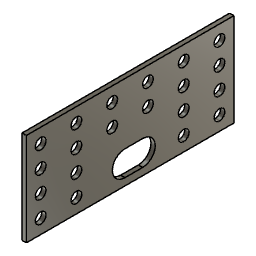
electronic_box_assembly v3 (Autodesk Fusion 360 archive; units mm, degrees)
design "plate_4"
Autodesk Fusion 360 part; units mm, degrees
sketch "Sketch1" plane through (0, 0, 0) normal (1, 0, 0) x (0, 1, 0)
  line L0 (0, 0) -> (290.2, 0)
  line L1 (290.2, 0) -> (290.2, 130)
  line L2 (290.2, 130) -> (0, 130)
  line L3 (0, 130) -> (0, 0)
  dimension "d1" = 290.2
  dimension "d2" = 130
  constraint horizontal L0
  constraint vertical L1
  constraint horizontal L2
  constraint vertical L3
  constraint coincident L0.start L3.end
  measures "d1" distance of L0.start L0.end
  measures "d2" distance of L0.start L2.end
extrude "Extrude1" add sketch "Sketch1" against normal blind 6
sketch "Sketch2" plane through (0, 0, 0) normal (1, 0, 0) x (0, 1, 0)
  line L0 (0, 130) -> (0, 0)
  line L1 (0, 0) -> (290.2, 0)
  line L2 (290.2, 0) -> (290.2, 130)
  line L3 (290.2, 130) -> (0, 130)
  line L4 (162.7, 45) -> (137.7, 45)
  arc A0 (137.7, 45) -> (137.7, 10) centre (137.7, 27.5) ccw
  line L5 (137.7, 10) -> (162.7, 10)
  arc A1 (162.7, 10) -> (162.7, 45) centre (162.7, 27.5) ccw
  line L6 (180.2, 27.5) -> (120.2, 27.5) construction
  circle A2 centre (20, 110) radius 7.5
  circle A3 centre (70, 110) radius 7.5
  circle A4 centre (120, 110) radius 7.5
  circle A5 centre (170, 110) radius 7.5
  circle A6 centre (220, 110) radius 7.5
  circle A7 centre (270, 110) radius 7.5
  circle A8 centre (20, 80) radius 7.5
  circle A9 centre (70, 80) radius 7.5
  circle A10 centre (120, 80) radius 7.5
  circle A11 centre (170, 80) radius 7.5
  circle A12 centre (220, 80) radius 7.5
  circle A13 centre (270, 80) radius 7.5
  circle A14 centre (20, 50) radius 7.5
  circle A15 centre (70, 50) radius 7.5
  circle A16 centre (220, 50) radius 7.5
  circle A17 centre (270, 50) radius 7.5
  circle A18 centre (20, 20) radius 7.5
  circle A19 centre (70, 20) radius 7.5
  circle A20 centre (220, 20) radius 7.5
  circle A21 centre (270, 20) radius 7.5
  dimension "d5" = 35
  dimension "d6" = 110
  dimension "d7" = 10
  dimension "d8" = 15
  dimension "d9" = 20
  dimension "d10" = 20
  dimension "d13" = 250
  dimension "d14" = -90
  constraint tangent L4 A0
  constraint tangent A0 L5
  constraint parallel L4 L5
  constraint tangent L5 A1
  constraint tangent L4 A1
  constraint midpoint A1 L6.start
  constraint midpoint A0 L6.end
  constraint horizontal L6
  measures "d5" diameter of A0
  measures "d6" distance of L2 L6.start
  measures "d7" distance of L1 L5
  measures "d8" diameter of A2
  measures "d9" distance of L3 A2.centre
  measures "d10" distance of L0 A2.centre
extrude "Extrude2" cut sketch "Sketch2" against normal up to surface (6 mm away) contours L4 A0 L5 A1 | A2 | A3 | A4 | A5 | A6 | A7 | A8 | A9 | A10 | A11 | A12 | A13 | A14 | A15 | A16 | A17 | A18 | A19 | A20 | A21

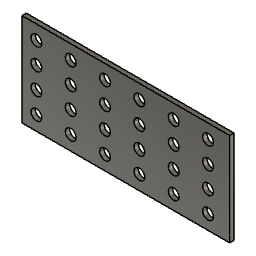
design "plate_2"
Autodesk Fusion 360 part; units mm, degrees
sketch "Sketch1" plane through (0, 0, 0) normal (0, 1, 0) x (1, 0, 0)
  line L0 (0, 0) -> (290.2, 0)
  line L1 (290.2, 0) -> (290.2, -130)
  line L2 (290.2, -130) -> (0, -130)
  line L3 (0, -130) -> (0, 0)
  dimension "d1" = 290.2
  dimension "d2" = 130
  constraint horizontal L0
  constraint vertical L1
  constraint horizontal L2
  constraint vertical L3
  constraint coincident L0.start L3.end
  measures "d1" distance of L0.start L0.end
  measures "d2" distance of L0.start L2.end
extrude "Extrude1" add sketch "Sketch1" against normal blind 6
sketch "Sketch2" plane through (0, -6, 0) normal (0, -1, 0) x (1, 0, 0)
  line L0 (290.2, 130) -> (0, 130)
  line L1 (0, 130) -> (0, 0)
  line L2 (0, 0) -> (290.2, 0)
  line L3 (290.2, 0) -> (290.2, 130)
  circle A0 centre (20, 110) radius 7.5
  circle A1 centre (68, 110) radius 7.5
  circle A2 centre (116, 110) radius 7.5
  circle A3 centre (164, 110) radius 7.5
  circle A4 centre (212, 110) radius 7.5
  circle A5 centre (260, 110) radius 7.5
  circle A6 centre (20, 80) radius 7.5
  circle A7 centre (68, 80) radius 7.5
  circle A8 centre (116, 80) radius 7.5
  circle A9 centre (164, 80) radius 7.5
  circle A10 centre (212, 80) radius 7.5
  circle A11 centre (260, 80) radius 7.5
  circle A12 centre (20, 50) radius 7.5
  circle A13 centre (68, 50) radius 7.5
  circle A14 centre (116, 50) radius 7.5
  circle A15 centre (164, 50) radius 7.5
  circle A16 centre (212, 50) radius 7.5
  circle A17 centre (260, 50) radius 7.5
  circle A18 centre (20, 20) radius 7.5
  circle A19 centre (68, 20) radius 7.5
  circle A20 centre (116, 20) radius 7.5
  circle A21 centre (164, 20) radius 7.5
  circle A22 centre (212, 20) radius 7.5
  circle A23 centre (260, 20) radius 7.5
  dimension "d5" = 15
  dimension "d6" = 20
  dimension "d7" = 20
  dimension "d10" = 240
  dimension "d11" = -90
  measures "d5" diameter of A0
  measures "d6" distance of L0 A0.centre
  measures "d7" distance of L1 A0.centre
extrude "Extrude2" cut sketch "Sketch2" against normal up to surface (6 mm away) contours A0 | A1 | A2 | A3 | A4 | A5 | A6 | A7 | A8 | A9 | A10 | A11 | A12 | A13 | A14 | A15 | A16 | A17 | A18 | A19 | A20 | A21 | A22 | A23

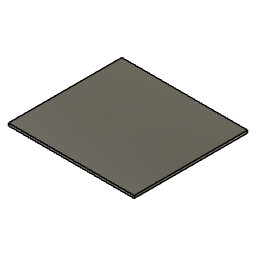
design "base_plate"
Autodesk Fusion 360 part; units mm, degrees
sketch "Sketch1" plane through (0, 0, 0) normal (0, 0, 1) x (1, 0, 0)
  line L0 (0, 0) -> (302.2, 0)
  line L1 (302.2, 0) -> (302.2, 272.2)
  line L2 (302.2, 272.2) -> (0, 272.2)
  line L3 (0, 272.2) -> (0, 0)
  dimension "d1" = 302.2
  dimension "d2" = 272.2
  constraint horizontal L0
  constraint vertical L1
  constraint horizontal L2
  constraint vertical L3
  constraint coincident L0.start L3.end
  measures "d1" distance of L0.start L0.end
  measures "d2" distance of L0 L2
extrude "Extrude1" add sketch "Sketch1" against normal blind 6

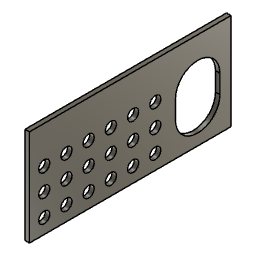
design "plate_1"
Autodesk Fusion 360 part; units mm, degrees
sketch "Sketch1" plane through (0, 0, 0) normal (1, 0, 0) x (0, 1, 0)
  line L0 (0, 0) -> (272.2, 0)
  line L1 (272.2, 0) -> (272.2, 130)
  line L2 (272.2, 130) -> (0, 130)
  line L3 (0, 130) -> (0, 0)
  dimension "d1" = 272.2
  dimension "d2" = 130
  constraint horizontal L0
  constraint vertical L1
  constraint horizontal L2
  constraint vertical L3
  constraint coincident L0.start L3.end
  measures "d1" distance of L0.start L0.end
  measures "d2" distance of L0.start L2.end
extrude "Extrude1" add sketch "Sketch1" against normal blind 6
sketch "Sketch2" plane through (0, 0, 0) normal (1, 0, 0) x (0, 1, 0)
  line L0 (0, 130) -> (0, 0)
  line L1 (0, 0) -> (272.2, 0)
  line L2 (272.2, 0) -> (272.2, 130)
  line L3 (272.2, 130) -> (0, 130)
  line L4 (257.2, 45) -> (257.2, 70)
  arc A0 (257.2, 70) -> (197.2, 70) centre (227.2, 70) ccw
  line L5 (197.2, 70) -> (197.2, 45)
  arc A1 (197.2, 45) -> (257.2, 45) centre (227.2, 45) ccw
  line L6 (227.2, 15) -> (227.2, 100) construction
  circle A2 centre (20, 80) radius 7.5
  circle A3 centre (50, 80) radius 7.5
  circle A4 centre (80, 80) radius 7.5
  circle A5 centre (110, 80) radius 7.5
  circle A6 centre (140, 80) radius 7.5
  circle A7 centre (170, 80) radius 7.5
  circle A8 centre (20, 50) radius 7.5
  circle A9 centre (50, 50) radius 7.5
  circle A10 centre (80, 50) radius 7.5
  circle A11 centre (110, 50) radius 7.5
  circle A12 centre (140, 50) radius 7.5
  circle A13 centre (170, 50) radius 7.5
  circle A14 centre (20, 20) radius 7.5
  circle A15 centre (50, 20) radius 7.5
  circle A16 centre (80, 20) radius 7.5
  circle A17 centre (110, 20) radius 7.5
  circle A18 centre (140, 20) radius 7.5
  circle A19 centre (170, 20) radius 7.5
  dimension "d5" = 60
  dimension "d6" = 15
  dimension "d7" = 15
  constraint tangent L4 A0
  constraint tangent A0 L5
  constraint parallel L4 L5
  constraint tangent L5 A1
  constraint tangent L4 A1
  constraint midpoint A1 L6.start
  constraint midpoint A0 L6.end
  constraint perpendicular L3 L6
  measures "d5" diameter of A0
  measures "d6" distance of L1 L6.start
  measures "d7" distance of L2 L4
extrude "Extrude2" cut sketch "Sketch2" against normal up to surface (6 mm away) contours L4 A0 L5 A1 | A2 | A3 | A4 | A5 | A6 | A7 | A8 | A9 | A10 | A11 | A12 | A13 | A14 | A15 | A16 | A17 | A18 | A19

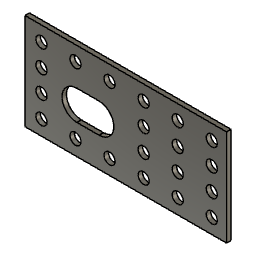
design "plate_3"
Autodesk Fusion 360 part; units mm, degrees
sketch "Sketch1" plane through (0, 0, 0) normal (0, 1, 0) x (1, 0, 0)
  line L0 (0, 0) -> (272.2, 0)
  line L1 (272.2, 0) -> (272.2, -130)
  line L2 (272.2, -130) -> (0, -130)
  line L3 (0, -130) -> (0, 0)
  dimension "d1" = 272.2
  dimension "d2" = 130
  constraint horizontal L0
  constraint vertical L1
  constraint horizontal L2
  constraint vertical L3
  constraint coincident L0.start L3.end
  measures "d1" distance of L0.start L0.end
  measures "d2" distance of L0.start L2.end
extrude "Extrude1" add sketch "Sketch1" against normal blind 6
sketch "Sketch2" plane through (0, -6, 0) normal (0, -1, 0) x (1, 0, 0)
  line L0 (272.2, 130) -> (0, 130)
  line L1 (0, 130) -> (0, 0)
  line L2 (0, 0) -> (272.2, 0)
  line L3 (272.2, 0) -> (272.2, 130)
  line L4 (70, 40) -> (100, 40)
  arc A0 (100, 40) -> (100, 80) centre (100, 60) ccw
  line L5 (100, 80) -> (70, 80)
  arc A1 (70, 80) -> (70, 40) centre (70, 60) ccw
  line L6 (50, 60) -> (120, 60) construction
  circle A2 centre (252.2, 110) radius 7.5
  circle A3 centre (206.2, 110) radius 7.5
  circle A4 centre (160.2, 110) radius 7.5
  circle A5 centre (114.2, 110) radius 7.5
  circle A6 centre (68.2, 110) radius 7.5
  circle A7 centre (252.2, 80) radius 7.5
  circle A8 centre (206.2, 80) radius 7.5
  circle A9 centre (252.2, 50) radius 7.5
  circle A10 centre (206.2, 50) radius 7.5
  circle A11 centre (160.2, 50) radius 7.5
  circle A12 centre (22.2, 110) radius 7.5
  circle A13 centre (22.2, 80) radius 7.5
  circle A14 centre (22.2, 50) radius 7.5
  circle A15 centre (252.2, 20) radius 7.5
  circle A16 centre (206.2, 20) radius 7.5
  circle A17 centre (160.2, 20) radius 7.5
  circle A18 centre (114.2, 20) radius 7.5
  circle A19 centre (68.2, 20) radius 7.5
  circle A20 centre (22.2, 20) radius 7.5
  circle A21 centre (160.2, 80) radius 7.5
  dimension "d5" = 40
  dimension "d6" = 50
  dimension "d8" = 40
  dimension "d9" = 15
  dimension "d10" = 20
  dimension "d11" = 20
  dimension "d14" = -230
  dimension "d15" = -90
  constraint tangent L4 A0
  constraint tangent A0 L5
  constraint parallel L4 L5
  constraint tangent L4 A1
  constraint midpoint A1 L6.start
  constraint midpoint A0 L6.end
  measures "d5" diameter of A0
  measures "d6" distance of L1 L6.start
  measures "d8" distance of L2 L4
  measures "d9" diameter of A2
  measures "d10" distance of L0 A2.centre
  measures "d11" distance of L3 A2.centre
extrude "Extrude2" cut sketch "Sketch2" against normal up to surface (6 mm away) contours L4 A0 L5 A1 | A2 | A3 | A4 | A5 | A6 | A7 | A8 | A9 | A10 | A11 | A12 | A13 | A14 | A15 | A16 | A17 | A18 | A19 | A20 | A21

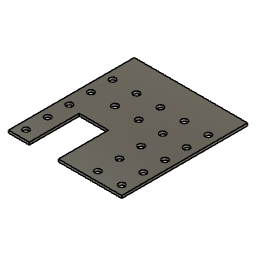
design "lid"
Autodesk Fusion 360 part; units mm, degrees
sketch "Sketch1" plane through (0, 0, 0) normal (0, 0, 1) x (1, 0, 0)
  line L0 (0, 0) -> (272.2, 0)
  line L1 (272.2, 0) -> (272.2, 302.2)
  line L2 (272.2, 302.2) -> (0, 302.2)
  line L3 (0, 302.2) -> (0, 0)
  dimension "d1" = 272.2
  dimension "d2" = 302.2
  constraint horizontal L0
  constraint vertical L1
  constraint horizontal L2
  constraint vertical L3
  constraint coincident L0.start L3.end
  measures "d1" distance of L0.start L0.end
  measures "d2" distance of L0.start L2.end
extrude "Extrude1" add sketch "Sketch1" against normal blind 6
sketch "Sketch2" plane through (0, 0, 0) normal (0, 0, 1) x (-1, 0, 0)
  line L0 (0, -302.2) -> (0, 0)
  line L1 (0, 0) -> (-272.2, 0)
  line L2 (-272.2, 0) -> (-272.2, -302.2)
  line L3 (-272.2, -302.2) -> (0, -302.2)
  line L4 (-50, 0) -> (-120, 0)
  line L5 (-120, 0) -> (-120, -120)
  line L6 (-120, -120) -> (-50, -120)
  line L7 (-50, -120) -> (-50, 0)
  circle A0 centre (-20, -230.2) radius 7.5
  circle A1 centre (-77.5, -230.2) radius 7.5
  circle A2 centre (-135, -230.2) radius 7.5
  circle A3 centre (-192.5, -230.2) radius 7.5
  circle A4 centre (-250, -230.2) radius 7.5
  circle A5 centre (-20, -178.2) radius 7.5
  circle A6 centre (-77.5, -178.2) radius 7.5
  circle A7 centre (-135, -178.2) radius 7.5
  circle A8 centre (-192.5, -178.2) radius 7.5
  circle A9 centre (-250, -178.2) radius 7.5
  circle A10 centre (-20, -126.2) radius 7.5
  circle A11 centre (-192.5, -126.2) radius 7.5
  circle A12 centre (-250, -126.2) radius 7.5
  circle A13 centre (-20, -74.2) radius 7.5
  circle A14 centre (-192.5, -74.2) radius 7.5
  circle A15 centre (-250, -74.2) radius 7.5
  circle A16 centre (-20, -22.2) radius 7.5
  circle A17 centre (-192.5, -22.2) radius 7.5
  circle A18 centre (-250, -22.2) radius 7.5
  dimension "d5" = 70
  dimension "d6" = 120
  dimension "d7" = 50
  constraint horizontal L4
  constraint vertical L5
  constraint horizontal L6
  constraint vertical L7
  constraint coincident L1 L4.start
  measures "d5" distance of L4.start L4.end
  measures "d6" distance of L4.start L6.end
  measures "d7" distance of L0 L7
extrude "Extrude2" cut sketch "Sketch2" against normal up to surface (6 mm away) contours L1 L4 L5 L6 L7 | A0 | A1 | A2 | A3 | A4 | A5 | A6 | A7 | A8 | A9 | A10 | A11 | A12 | A13 | A14 | A15 | A16 | A17 | A18
